Autodesk Fusion 360 part; units mm, degrees
(part 2 of 2)
sketch "Voronoi Sketch (1)" plane through (0, 0, 0) normal (0, 1, 0) x (1, 0, 0)
  line L0 (-147.4553, 380.9764) -> (-22.91, 349.763)
  line L1 (-20, 352.0337) -> (-20, 415.577)
  line L2 (-22.9871, 418.299) -> (-142.016, 407.2223)
  line L3 (-145.6266, 404.0099) -> (-149.7418, 384.6402)
  line L4 (-186.1493, 320.3463) -> (-22.796, 256.8129)
  line L5 (-20, 258.7255) -> (-20, 325.4152)
  line L6 (-22.91, 329.1445) -> (-155.1899, 362.2963)
  line L7 (-159.887, 360.616) -> (-187.1582, 323.8434)
  line L8 (-22.0935, 215.5532) -> (-62.0213, 174.5726)
  line L9 (-61.6187, 170.7597) -> (-22.4961, 144.6769)
  line L10 (-20, 146.0128) -> (-20, 214.7019)
  line L11 (-476.2673, 20) -> (-393.481, 20)
  line L12 (-391.1606, 22.922) -> (-411.0139, 108.2903)
  line L13 (-414.2696, 112.7498) -> (-436.7994, 126.1956)
  line L14 (-440.4173, 124.9197) -> (-478.2255, 22.8133)
  line L15 (-366.3033, 260.6743) -> (-336.0165, 355.7495)
  line L16 (-337.6139, 360.2543) -> (-347.7063, 366.8791)
  line L17 (-351.256, 365.712) -> (-388.3314, 265.5847)
  line L18 (-386.4455, 262.1166) -> (-370.1416, 258.4705)
  line L19 (-305.95, 488.0669) -> (-342.046, 390.5847)
  line L20 (-340.5798, 386.1251) -> (-321.3476, 373.5007)
  line L21 (-316.0018, 370.8814) -> (-208.1565, 333.9038)
  line L22 (-203.5316, 335.3404) -> (-173.2675, 376.1486)
  line L23 (-170.857, 381.4927) -> (-163.9276, 414.1079)
  line L24 (-163.4419, 420.0392) -> (-166.0427, 476.6123)
  line L25 (-168.9703, 480.7121) -> (-247.2406, 511.6581)
  line L26 (-253.0159, 513.0559) -> (-290.3514, 516.7429)
  line L27 (-296.0199, 515.6955) -> (-296.8408, 515.2849)
  arc A0 (-305.95, 488.0669) -> (-299.907, 511.1034) centre (-419.9835, 530.2916) ccw
  line L28 (-306.3425, 576.2843) -> (-308.6586, 678.37)
  line L29 (-311.4233, 680.0548) -> (-367.5134, 652.7162)
  line L30 (-368.0562, 649.3136) -> (-335.342, 617.5979)
  arc A1 (-307.3333, 576.079) -> (-335.342, 617.5979) centre (-419.9835, 530.2916) ccw
  line L31 (-290.1367, 792.8) -> (-513.06, 792.8)
  line L32 (-513.9061, 790.7118) -> (-387.6359, 668.2956)
  line L33 (-382.7852, 667.5218) -> (-308.1936, 703.8782)
  line L34 (-303.6279, 707.5393) -> (-292.5089, 721.5008)
  line L35 (-290.4877, 726.8437) -> (-287.2889, 789.8039)
  line L36 (-31.3886, 792.8) -> (-264.1109, 792.8)
  line L37 (-267.2631, 789.8039) -> (-270.425, 727.5711)
  line L38 (-268.2847, 722.6399) -> (-210.4667, 673.8356)
  line L39 (-205.4064, 670.7434) -> (-152.3507, 648.5628)
  line L40 (-147.662, 649.71) -> (-30.3094, 790.4956)
  line L41 (-281.2725, 703.506) -> (-287.1345, 696.1453)
  line L42 (-288.9354, 690.7994) -> (-285.4995, 539.3535)
  line L43 (-282.446, 536.0595) -> (-258.3048, 533.6755)
  line L44 (-254.6106, 536.2958) -> (-225.3372, 656.702)
  line L45 (-226.921, 661.5521) -> (-277.111, 703.9176)
  line L46 (-20, 23) -> (-20, 115.9754)
  line L47 (-22.4961, 120.6396) -> (-78.8526, 158.2122)
  line L48 (-84.2287, 159.0361) -> (-95.8589, 155.6433)
  line L49 (-99.6958, 151.9598) -> (-127.0602, 70.6513)
  line L50 (-127.0367, 64.9728) -> (-112.4656, 22.8353)
  line L51 (-108.4852, 20) -> (-23, 20)
  line L52 (-299.6469, 20) -> (-135.6472, 20)
  line L53 (-133.6276, 22.8353) -> (-145.6876, 57.711)
  line L54 (-149.3744, 61.8406) -> (-198.8564, 85.5062)
  line L55 (-204.4375, 87.6585) -> (-259.148, 103.9843)
  line L56 (-263.3183, 102.1363) -> (-301.3513, 22.7058)
  line L57 (-192.6305, 298.3037) -> (-193.4348, 290.5107)
  line L58 (-192.05, 285.0498) -> (-178.0594, 264.5796)
  line L59 (-174.4432, 259.8006) -> (-104.995, 176.6751)
  line L60 (-100.1916, 175.213) -> (-87.8837, 178.8035)
  line L61 (-82.9102, 181.7924) -> (-30.6397, 235.4412)
  line L62 (-31.3422, 238.6774) -> (-189.5265, 300.2004)
  line L63 (-184.6975, 100.9042) -> (-147.1643, 82.9533)
  line L64 (-143.501, 84.5022) -> (-118.7713, 157.9819)
  line L65 (-119.7379, 163.1274) -> (-174.5225, 228.7014)
  line L66 (-176.7002, 228.0145) -> (-187.1496, 105.1878)
  line L67 (-336.0997, 142.0941) -> (-388.7978, 113.8426)
  line L68 (-390.7623, 109.5032) -> (-370.6268, 22.922)
  line L69 (-366.9473, 20) -> (-327.8214, 20)
  line L70 (-323.5258, 22.7058) -> (-279.6279, 114.3851)
  line L71 (-279.517, 119.8471) -> (-285.9338, 134.7746)
  line L72 (-290.0939, 137.9148) -> (-330.4803, 143.1275)
  line L73 (-400.0087, 130.5252) -> (-351.4194, 156.574)
  line L74 (-350.1571, 160.6543) -> (-365.7248, 190.6572)
  line L75 (-370.1, 193.1224) -> (-413.2987, 190.2705)
  line L76 (-417.3339, 187.2595) -> (-431.2705, 149.6219)
  line L77 (-429.7361, 145.2712) -> (-405.2288, 130.6452)
  line L78 (-368.4843, 216.1382) -> (-364.7953, 231.1183)
  line L79 (-368.9276, 237.705) -> (-393.4537, 243.1899)
  line L80 (-397.4231, 241.0313) -> (-407.6427, 213.432)
  line L81 (-405.6909, 210.8163) -> (-372.1952, 213.0276)
  line L82 (-346.8257, 245.3081) -> (-249.9731, 248.4399)
  line L83 (-245.0675, 250.8526) -> (-215.6107, 286.621)
  line L84 (-213.3955, 291.921) -> (-211.447, 310.7993)
  line L85 (-213.9769, 314.7565) -> (-314.0108, 349.0558)
  line L86 (-317.7592, 347.1703) -> (-349.125, 248.7079)
  line L87 (-268.1456, 144.0367) -> (-261.1961, 127.8695)
  line L88 (-257.1366, 124.2555) -> (-209.7504, 110.1153)
  line L89 (-206.6213, 112.2467) -> (-194.8705, 250.3708)
  line L90 (-196.309, 255.8368) -> (-203.1173, 265.7983)
  line L91 (-206.7172, 265.9593) -> (-231.5546, 235.8003)
  line L92 (-234.6087, 230.7124) -> (-268.1834, 149.5649)
  line L93 (-260.2939, 228.0957) -> (-342.6231, 225.4336)
  line L94 (-346.3389, 222.4236) -> (-349.9141, 207.9061)
  line L95 (-349.2497, 202.3303) -> (-330.2694, 165.7508)
  line L96 (-325.9124, 162.7039) -> (-289.4717, 158.0004)
  line L97 (-285.3495, 160.3885) -> (-258.4425, 225.4206)
  line L98 (-146.1848, 480.163) -> (-143.8853, 430.1444)
  line L99 (-140.7605, 427.4256) -> (-22.9871, 438.3854)
  line L100 (-20, 441.6634) -> (-20, 447.4329)
  line L101 (-22.5271, 452.0497) -> (-117.9512, 513.0987)
  line L102 (-122.3792, 512.3945) -> (-144.4217, 485.4808)
  line L103 (-233.0913, 527.5703) -> (-162.3893, 499.6166)
  line L104 (-157.6986, 500.8345) -> (-132.7542, 531.2913)
  line L105 (-129.37, 536.2199) -> (-127.7214, 539.1182)
  line L106 (-127.1791, 544.5744) -> (-153.7523, 625.0161)
  line L107 (-157.4612, 629.0219) -> (-203.7321, 648.366)
  line L108 (-207.2087, 646.6081) -> (-235.1724, 531.5884)
  line L109 (-21.9209, 769.3231) -> (-133.4703, 635.4995)
  line L110 (-134.4501, 630.3464) -> (-109.8687, 555.9343)
  line L111 (-106.0607, 553.969) -> (-103.9618, 554.6156)
  line L112 (-99.8422, 558.2249) -> (-21.2525, 729.2702)
  line L113 (-20, 734.9962) -> (-20, 768.6275)
  line L114 (-21.2525, 681.3667) -> (-76.0488, 562.1062)
  line L115 (-74.3239, 559.7476) -> (-22.9774, 566.0835)
  line L116 (-20, 569.4509) -> (-20, 681.0927)
  line L117 (-108.7023, 530.9243) -> (-22.5271, 475.7925)
  line L118 (-20, 477.1757) -> (-20, 543.2992)
  line L119 (-22.9774, 545.9318) -> (-88.7974, 537.81)
  line L120 (-94.6419, 536.5593) -> (-108.0588, 532.4258)
  arc A2 (-142.016, 407.2223) -> (-145.6266, 404.0099) centre (-141.6382, 403.1625) ccw
  arc A3 (-149.7418, 384.6402) -> (-147.4553, 380.9764) centre (-146.6991, 383.9938) ccw
  arc A4 (-20, 415.577) -> (-22.9871, 418.299) centre (-22.7338, 415.577) ccw
  arc A5 (-22.91, 349.763) -> (-20, 352.0337) centre (-22.3409, 352.0337) ccw
  arc A6 (-155.1899, 362.2963) -> (-159.887, 360.616) centre (-156.2812, 357.9419) ccw
  arc A7 (-20, 325.4152) -> (-22.91, 329.1445) centre (-23.8446, 325.4152) ccw
  arc A8 (-187.1582, 323.8434) -> (-186.1493, 320.3463) centre (-185.3195, 322.4798) ccw
  arc A9 (-22.796, 256.8129) -> (-20, 258.7255) centre (-22.0521, 258.7255) ccw
  arc A10 (-22.4961, 144.6769) -> (-20, 146.0128) centre (-21.6055, 146.0128) ccw
  arc A11 (-20, 214.7019) -> (-22.0935, 215.5532) centre (-21.2198, 214.7019) ccw
  arc A12 (-62.0213, 174.5726) -> (-61.6187, 170.7597) centre (-60.2362, 172.8334) ccw
  arc A13 (-411.0139, 108.2903) -> (-414.2696, 112.7498) centre (-417.8846, 106.6925) ccw
  arc A14 (-436.7994, 126.1956) -> (-440.4173, 124.9197) centre (-438.0779, 124.0535) ccw
  arc A15 (-478.2255, 22.8133) -> (-476.2673, 20) centre (-476.2673, 22.0882) ccw
  arc A16 (-393.481, 20) -> (-391.1606, 22.922) centre (-393.481, 22.3824) ccw
  arc A17 (-336.0165, 355.7495) -> (-337.6139, 360.2543) centre (-339.7833, 356.9495) ccw
  arc A18 (-388.3314, 265.5847) -> (-386.4455, 262.1166) centre (-385.8734, 264.6745) ccw
  arc A19 (-347.7063, 366.8791) -> (-351.256, 365.712) centre (-349.0166, 364.8829) ccw
  arc A20 (-370.1416, 258.4705) -> (-366.3033, 260.6743) centre (-369.4263, 261.6691) ccw
  arc A21 (-290.3514, 516.7429) -> (-296.0199, 515.6955) centre (-291.3723, 506.4048) ccw
  arc A22 (-296.8408, 515.2849) -> (-299.907, 511.1034) centre (-294.3009, 510.2075) ccw
  arc A23 (-342.046, 390.5847) -> (-340.5798, 386.1251) centre (-338.5115, 389.2759) ccw
  arc A24 (-173.2675, 376.1486) -> (-170.857, 381.4927) centre (-184.3346, 384.3562) ccw
  arc A25 (-321.3476, 373.5007) -> (-316.0018, 370.8814) centre (-308.2757, 393.4146) ccw
  arc A26 (-163.9276, 414.1079) -> (-163.4419, 420.0392) centre (-186.7925, 418.9658) ccw
  arc A27 (-247.2406, 511.6581) -> (-253.0159, 513.0559) centre (-255.1226, 491.7224) ccw
  arc A28 (-208.1565, 333.9038) -> (-203.5316, 335.3404) centre (-206.8261, 337.7837) ccw
  arc A29 (-166.0427, 476.6123) -> (-168.9703, 480.7121) centre (-170.6755, 476.3993) ccw
  arc A30 (-367.5134, 652.7162) -> (-368.0562, 649.3136) centre (-366.5914, 650.8245) ccw
  arc A31 (-307.3333, 576.079) -> (-306.3425, 576.2843) centre (-306.8567, 576.2727) ccw
  arc A32 (-308.6586, 678.37) -> (-311.4233, 680.0548) centre (-310.5809, 678.3264) ccw
  arc A33 (-308.1936, 703.8782) -> (-303.6279, 707.5393) centre (-314.0069, 715.8051) ccw
  arc A34 (-292.5089, 721.5008) -> (-290.4877, 726.8437) centre (-299.8125, 727.3174) ccw
  arc A35 (-287.2889, 789.8039) -> (-290.1367, 792.8) centre (-290.1367, 789.9486) ccw
  arc A36 (-387.6359, 668.2956) -> (-382.7852, 667.5218) centre (-384.659, 671.3662) ccw
  arc A37 (-513.06, 792.8) -> (-513.9061, 790.7118) centre (-513.06, 791.5845) ccw
  arc A38 (-210.4667, 673.8356) -> (-205.4064, 670.7434) centre (-197.8795, 688.7476) ccw
  arc A39 (-264.1109, 792.8) -> (-267.2631, 789.8039) centre (-264.1109, 789.6437) ccw
  arc A40 (-152.3507, 648.5628) -> (-147.662, 649.71) centre (-150.7833, 652.3119) ccw
  arc A41 (-270.425, 727.5711) -> (-268.2847, 722.6399) centre (-264.3815, 727.264) ccw
  arc A42 (-30.3094, 790.4956) -> (-31.3886, 792.8) centre (-31.3886, 791.3951) ccw
  arc A43 (-277.111, 703.9176) -> (-281.2725, 703.506) centre (-278.9917, 701.6896) ccw
  arc A44 (-287.1345, 696.1453) -> (-288.9354, 690.7994) centre (-280.6577, 690.9872) ccw
  arc A45 (-258.3048, 533.6755) -> (-254.6106, 536.2958) centre (-257.9655, 537.1114) ccw
  arc A46 (-285.4995, 539.3535) -> (-282.446, 536.0595) centre (-282.1131, 539.4304) ccw
  arc A47 (-225.3372, 656.702) -> (-226.921, 661.5521) centre (-230.0482, 657.8473) ccw
  arc A48 (-95.8589, 155.6433) -> (-99.6958, 151.9598) centre (-94.2496, 150.1269) ccw
  arc A49 (-78.8526, 158.2122) -> (-84.2287, 159.0361) centre (-82.4251, 152.8537) ccw
  arc A50 (-127.0602, 70.6513) -> (-127.0367, 64.9728) centre (-118.7262, 67.8465) ccw
  arc A51 (-112.4656, 22.8353) -> (-108.4852, 20) centre (-108.4852, 24.2117) ccw
  arc A52 (-23, 20) -> (-20, 23) centre (-23, 23) ccw
  arc A53 (-20, 115.9754) -> (-22.4961, 120.6396) centre (-25.6057, 115.9754) ccw
  arc A54 (-135.6472, 20) -> (-133.6276, 22.8353) centre (-135.6472, 22.1369) ccw
  arc A55 (-198.8564, 85.5062) -> (-204.4375, 87.6585) centre (-215.4047, 50.9057) ccw
  arc A56 (-145.6876, 57.711) -> (-149.3744, 61.8406) centre (-152.4714, 55.3651) ccw
  arc A57 (-259.148, 103.9843) -> (-263.3183, 102.1363) centre (-260.1519, 100.6202) ccw
  arc A58 (-301.3513, 22.7058) -> (-299.6469, 20) centre (-299.6469, 21.8897) ccw
  arc A59 (-189.5265, 300.2004) -> (-192.6305, 298.3037) centre (-190.3555, 298.0689) ccw
  arc A60 (-104.995, 176.6751) -> (-100.1916, 175.213) centre (-101.4758, 179.6152) ccw
  arc A61 (-193.4348, 290.5107) -> (-192.05, 285.0498) centre (-185.2899, 289.6701) ccw
  arc A62 (-87.8837, 178.8035) -> (-82.9102, 181.7924) centre (-91.0769, 189.7493) ccw
  arc A63 (-178.0594, 264.5796) -> (-174.4432, 259.8006) centre (-126.7422, 299.653) ccw
  arc A64 (-30.6397, 235.4412) -> (-31.3422, 238.6774) centre (-32.0619, 236.8269) ccw
  arc A65 (-187.1496, 105.1878) -> (-184.6975, 100.9042) centre (-182.8248, 104.8199) ccw
  arc A66 (-118.7713, 157.9819) -> (-119.7379, 163.1274) centre (-123.8507, 159.6913) ccw
  arc A67 (-147.1643, 82.9533) -> (-143.501, 84.5022) centre (-146.0183, 85.3494) ccw
  arc A68 (-174.5225, 228.7014) -> (-176.7002, 228.0145) centre (-175.47, 227.9098) ccw
  arc A69 (-279.6279, 114.3851) -> (-279.517, 119.8471) centre (-285.5863, 117.2381) ccw
  arc A70 (-285.9338, 134.7746) -> (-290.0939, 137.9148) centre (-290.7673, 132.6969) ccw
  arc A71 (-327.8214, 20) -> (-323.5258, 22.7058) centre (-327.8214, 24.7626) ccw
  arc A72 (-330.4803, 143.1275) -> (-336.0997, 142.0941) centre (-331.6782, 133.8467) ccw
  arc A73 (-370.6268, 22.922) -> (-366.9473, 20) centre (-366.9473, 23.7777) ccw
  arc A74 (-388.7978, 113.8426) -> (-390.7623, 109.5032) centre (-386.9471, 110.3904) ccw
  arc A75 (-431.2705, 149.6219) -> (-429.7361, 145.2712) centre (-427.8872, 148.3692) ccw
  arc A76 (-351.4194, 156.574) -> (-350.1571, 160.6543) centre (-352.856, 159.2539) ccw
  arc A77 (-413.2987, 190.2705) -> (-417.3339, 187.2595) centre (-412.9938, 185.6525) ccw
  arc A78 (-405.2288, 130.6452) -> (-400.0087, 130.5252) centre (-402.5128, 135.1962) ccw
  arc A79 (-365.7248, 190.6572) -> (-370.1, 193.1224) centre (-369.7978, 188.5438) ccw
  arc A80 (-365.4717, 235.2727) -> (-368.9276, 237.705) centre (-370.131, 232.3238) ccw
  arc A81 (-364.7953, 231.1183) -> (-365.4717, 235.2727) centre (-370.0076, 232.4019) ccw
  arc A82 (-393.4537, 243.1899) -> (-397.4231, 241.0313) centre (-394.2031, 239.8389) ccw
  arc A83 (-372.1952, 213.0276) -> (-368.4843, 216.1382) centre (-372.4652, 217.1186) ccw
  arc A84 (-407.6427, 213.432) -> (-405.6909, 210.8163) centre (-405.819, 212.7567) ccw
  arc A85 (-348.8238, 246.3665) -> (-346.8257, 245.3081) centre (-346.8993, 247.5845) ccw
  arc A86 (-349.125, 248.7079) -> (-348.8238, 246.3665) centre (-346.4638, 247.8602) ccw
  arc A87 (-215.6107, 286.621) -> (-213.3955, 291.921) centre (-223.2857, 292.9417) ccw
  arc A88 (-211.447, 310.7993) -> (-213.9769, 314.7565) centre (-215.2008, 311.1867) ccw
  arc A89 (-249.9731, 248.4399) -> (-245.0675, 250.8526) centre (-250.1875, 255.0691) ccw
  arc A90 (-314.0108, 349.0558) -> (-317.7592, 347.1703) centre (-314.9628, 346.2795) ccw
  arc A91 (-194.8705, 250.3708) -> (-196.309, 255.8368) centre (-203.262, 251.0847) ccw
  arc A92 (-268.1834, 149.5649) -> (-268.1456, 144.0367) centre (-261.6111, 146.8456) ccw
  arc A93 (-203.1173, 265.7983) -> (-206.7172, 265.9593) centre (-204.9778, 264.5268) ccw
  arc A94 (-261.1961, 127.8695) -> (-257.1366, 124.2555) centre (-255.3021, 130.4031) ccw
  arc A95 (-231.5546, 235.8003) -> (-234.6087, 230.7124) centre (-216.0554, 223.036) ccw
  arc A96 (-209.7504, 110.1153) -> (-206.6213, 112.2467) centre (-209.0526, 112.4535) ccw
  arc A97 (-349.9141, 207.9061) -> (-349.2497, 202.3303) centre (-342.1762, 206.0006) ccw
  arc A98 (-342.6231, 225.4336) -> (-346.3389, 222.4236) centre (-342.4952, 221.4771) ccw
  arc A99 (-330.2694, 165.7508) -> (-325.9124, 162.7039) centre (-325.1782, 168.3925) ccw
  arc A100 (-289.4717, 158.0004) -> (-285.3495, 160.3885) centre (-288.9702, 161.8865) ccw
  arc A101 (-258.4425, 225.4206) -> (-260.2939, 228.0957) centre (-260.2314, 226.1608) ccw
  arc A102 (-20, 447.4329) -> (-22.5271, 452.0497) centre (-25.4807, 447.4329) ccw
  arc A103 (-22.9871, 438.3854) -> (-20, 441.6634) centre (-23.2921, 441.6634) ccw
  arc A104 (-117.9512, 513.0987) -> (-122.3792, 512.3945) centre (-119.7692, 510.257) ccw
  arc A105 (-144.4217, 485.4808) -> (-146.1848, 480.163) centre (-138.3676, 480.5224) ccw
  arc A106 (-143.8853, 430.1444) -> (-140.7605, 427.4256) centre (-141.0257, 430.2759) ccw
  arc A107 (-127.7214, 539.1182) -> (-127.1791, 544.5744) centre (-133.5902, 542.4566) ccw
  arc A108 (-132.7542, 531.2913) -> (-129.37, 536.2199) centre (-160.1491, 553.728) ccw
  arc A109 (-153.7523, 625.0161) -> (-157.4612, 629.0219) centre (-159.9984, 622.9528) ccw
  arc A110 (-235.1724, 531.5884) -> (-233.0913, 527.5703) centre (-231.8244, 530.7745) ccw
  arc A111 (-162.3893, 499.6166) -> (-157.6986, 500.8345) centre (-160.8782, 503.4386) ccw
  arc A112 (-203.7321, 648.366) -> (-207.2087, 646.6081) centre (-204.72, 646.003) ccw
  arc A113 (-109.8687, 555.9343) -> (-106.0607, 553.969) centre (-106.962, 556.8945) ccw
  arc A114 (-103.9618, 554.6156) -> (-99.8422, 558.2249) centre (-105.9364, 561.025) ccw
  arc A115 (-21.2525, 729.2702) -> (-20, 734.9962) centre (-33.7148, 734.9962) ccw
  arc A116 (-20, 768.6275) -> (-21.9209, 769.3231) centre (-21.0864, 768.6275) ccw
  arc A117 (-133.4703, 635.4995) -> (-134.4501, 630.3464) centre (-129.321, 632.0408) ccw
  arc A118 (-22.9774, 566.0835) -> (-20, 569.4509) centre (-23.3929, 569.4509) ccw
  arc A119 (-76.0488, 562.1062) -> (-74.3239, 559.7476) centre (-74.5287, 561.4078) ccw
  arc A120 (-20, 681.0927) -> (-21.2525, 681.3667) centre (-20.6562, 681.0927) ccw
  arc A121 (-108.0588, 532.4258) -> (-108.9054, 531.7464) centre (-107.6251, 531.0182) ccw
  arc A122 (-108.9054, 531.7464) -> (-108.7023, 530.9243) centre (-108.3708, 531.4423) ccw
  arc A123 (-88.7974, 537.81) -> (-94.6419, 536.5593) centre (-84.6352, 504.0789) ccw
  arc A124 (-22.5271, 475.7925) -> (-20, 477.1757) centre (-21.6421, 477.1757) ccw
  arc A125 (-20, 543.2992) -> (-22.9774, 545.9318) centre (-22.6526, 543.2992) ccw
  line L121 (0, 0) -> (0, 812.8)
  line L122 (0, 812.8) -> (-565.2203, 812.8)
  arc A126 (-565.2203, 812.8) -> (-561.4783, 808.976) centre (-490.7581, 881.9227) ccw
  line L123 (-561.4783, 808.976) -> (-349.2633, 603.2383)
  arc A127 (-324.7055, 495.0118) -> (-349.2633, 603.2383) centre (-419.9835, 530.2916) ccw
  line L124 (-324.7055, 495.0118) -> (-508, 0)
  line L125 (-508, 0) -> (0, 0)
sketch "Voronoi Sites Sketch (1)" plane through (0, 0, 0) normal (0, 1, 0) x (1, 0, 0)
  point P0 (-449.0524, 72.9621)
  point P1 (-86.3037, 237.1655)
  point P2 (-70.5539, 636.8662)
  point P3 (-41.0771, 623.3225)
  point P4 (-235.4425, 46.9716)
  point P5 (-250.7806, 601.4917)
  point P6 (-24.1707, 486.3122)
  point P7 (-43.5453, 456.0282)
  point P8 (-403.1679, 722.8538)
  point P9 (-266.1559, 445.7943)
  point P10 (-49.5694, 111.2462)
  point P11 (-63.5895, 295.5671)
  point P12 (-158.818, 710.4391)
  point P13 (-341.81, 97.9025)
  point P14 (-376.7004, 277.3889)
  point P15 (-327.3953, 209.5826)
  point P16 (-208.6473, 591.2482)
  point P17 (-13.1427, 165.884)
  point P18 (-329.0975, 262.2247)
  point P19 (-38.0837, 397.3382)
  point P20 (-385.5146, 179.4258)
  point P21 (-388.499, 224.6302)
  point P22 (-342.9956, 599.3996)
  point P23 (-202.3565, 157.8478)
  point P24 (-183.1936, 156.2176)
extrude "Extrude3" add sketch "Voronoi Sketch (1)" along normal blind 12.7 makes body 1
extrude "Extrude4" add sketch "Voronoi Sketch" along normal blind 12.7 separate body makes body 2
